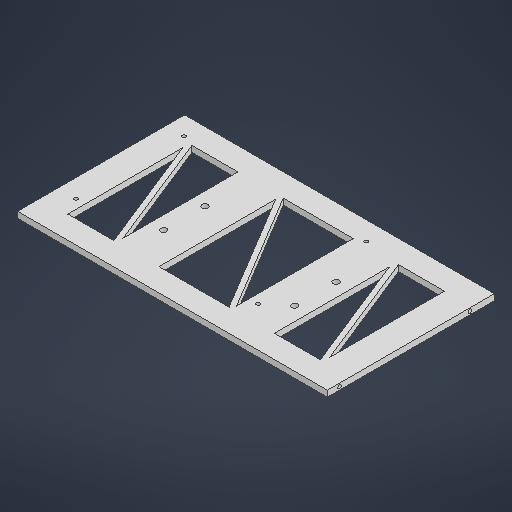
# Autodesk Inventor part: midplate
Saved by Autodesk Inventor 2025.1 (Build 291241000, 241)
## iProperties
Created: 2025-03-19
Part Number: midplate
Material: Generic
Document SubType Name: Modeling
Designer: m_kni
Density: 1 g/cm^3
Appearance: Default
Author: m_kni
## iProperties of the stored document midplate_3DPrint.ipt
Created: 2025-03-27
Part Number: midplate_3DPrint
Material: Generic
Document SubType Name: Modeling
Designer: jerem
Density: 1 g/cm^3
Appearance: Default
Author: jerem
Autodesk Inventor part; units mm, degrees
ref_plane "YZ Plane" through (0, 0, 0) normal (1, 0, 0) x (0, 1, 0)
ref_plane "XZ Plane" through (0, 0, 0) normal (0, 1, 0) x (-1, 0, 0)
ref_plane "XY Plane" through (0, 0, 0) normal (0, 0, 1) x (1, 0, 0)
sketch "Sketch1" plane through (0, 0, 0) normal (0, 1, 0) x (-1, 0, 0)
  circle A0 centre (-37.3734, -58.1709) radius 1.5
  circle A1 centre (112.6266, 30.8291) radius 1.5
  circle A2 centre (-37.3734, 30.8291) radius 1.5
  circle A3 centre (112.6266, -58.1709) radius 1.5
  circle A4 centre (54.1266, -16.9209) radius 2.5
  circle A5 centre (-53.8734, 17.0791) radius 2.5
  circle A6 centre (54.1266, 17.0791) radius 2.5
  circle A7 centre (-53.8734, -16.9209) radius 2.5
  line L0 (-127.3734, 73.8291) -> (127.6266, 73.8291)
  line L1 (-127.3734, -73.6709) -> (-127.3734, 73.8291)
  line L2 (127.6266, -73.6709) -> (-127.3734, -73.6709)
  line L3 (127.6266, 73.8291) -> (127.6266, -73.6709)
  point P0 (0, 0)
  point P1 (0.1266, 73.8291)
  constraints: 8 centre point, 8 end point
extrude "Extrusion1" add sketch "Sketch1" along normal blind 10
sketch "Sketch2" plane through (127.3734, 0, 73.8291) normal (1, 0, 0) x (0, 0, -1)
  line L0 (147.5, 0) -> (147.5, 10) projected
  line L1 (0, 0) -> (0, 10) projected
  circle A0 centre (127.5, 5) radius 1.5
  circle A1 centre (20, 5) radius 1.5
  point P0 (73.8291, 0)
  point P1 (0, 5)
  dimension "d2" = 20
  dimension "d3" = 20
  dimension "d4" = 3
  dimension "d5" = 3
  constraints: 2 centre point, 2 coincident, 1 midpoint
  measures "d2" distance from line of point (127.5, 5) L0
  measures "d3" distance of point (20, 5) point (0, 5)
  measures "d4" diameter of A0
  measures "d5" diameter of A1
extrude "Extrusion2" cut sketch "Sketch2" against normal blind 6
ref_plane "Work Plane1" through (-0.1266, 0, 73.8291) normal (1, 0, 0) x (0, 0, -1)
mirror "Mirror1" about plane through (-0.1266, 0, 73.8291) normal (1, 0, 0) of "Extrusion2"
sketch "Sketch3" plane through (-127.6266, 0, 73.8291) normal (0, 0, 1) x (1, 0, 0)
  line L0 (255, 10) -> (0, 10) projected
  line L1 (255, 0) -> (0, 0)
  line L2 (0, 0) -> (0, 10)
  line L3 (0, 10) -> (255, 10)
  line L4 (255, 10) -> (255, 0)
  point P0 (127.6266, 0)
  constraints: 8 end point, 2 parallel, 1 horizontal, 1 perpendicular
extrude "Extrusion3" cut sketch "Sketch3" against normal blind 10
sketch "Sketch4" plane through (0, 10, 0) normal (0, 1, 0) x (1, 0, 0)
  line L0 (127.3734, -63.8291) -> (127.3734, 73.6709) projected
  line L1 (-127.6266, -63.8291) -> (127.3734, -63.8291)
  line L2 (127.3734, -63.8291) -> (127.3734, 73.6709)
  line L3 (127.3734, 73.6709) -> (-127.6266, 73.6709)
  line L4 (-127.6266, 73.6709) -> (-127.6266, -63.8291)
  point P0 (0, 0)
  constraints: 8 end point, 2 parallel, 1 horizontal, 1 perpendicular
ref_plane "Work Plane2" through (0, 5, 0) normal (0, 1, 0) x (1, 0, 0)
extrude "Extrusion4" cut sketch "Sketch4" against normal blind 2.5
mirror "Mirror2" about plane through (0, 5, 0) normal (0, 1, 0) of "Extrusion4"
sketch "Sketch6" plane through (0, 7.5, 0) normal (0, 1, 0) x (1, 0, 0)
  circle A0 centre (37.3734, 58.1709) radius 1.5 projected
  circle A1 centre (-112.6266, -30.8291) radius 1.5 projected
  circle A2 centre (37.3734, -30.8291) radius 1.5 projected
  circle A3 centre (-112.6266, 58.1709) radius 1.5 projected
  circle A4 centre (-54.1266, 16.9209) radius 2.5 projected
  circle A5 centre (53.8734, -17.0791) radius 2.5 projected
  circle A6 centre (-54.1266, -17.0791) radius 2.5 projected
  circle A7 centre (53.8734, 16.9209) radius 2.5 projected
  line L0 (127.3734, 73.6709) -> (127.3734, -63.8291) projected
  line L1 (-127.6266, 73.6709) -> (127.3734, 73.6709) projected
  line L2 (-127.6266, -63.8291) -> (-127.6266, 73.6709) projected
  line L3 (127.3734, -63.8291) -> (-127.6266, -63.8291) projected
  line L4 (-30, 54.9209) -> (30, 54.9209)
  line L5 (30, 54.9209) -> (30, -45.0791)
  line L6 (30, -45.0791) -> (-30, -45.0791)
  line L7 (-30, -45.0791) -> (-30, 54.9209)
  line L8 (-105, 54.9209) -> (-65, 54.9209)
  line L9 (-65, 54.9209) -> (-65, -45.0791)
  line L10 (-65, -45.0791) -> (-105, -45.0791)
  line L11 (-105, -45.0791) -> (-105, 54.9209)
  line L12 (65, 54.9209) -> (105, 54.9209)
  line L13 (105, 54.9209) -> (105, -45.0791)
  line L14 (105, -45.0791) -> (65, -45.0791)
  line L15 (65, -45.0791) -> (65, 54.9209)
  line L16 (-65, 4.9209) -> (-30, 4.9209) construction
  line L17 (30, 4.9209) -> (65, 4.9209) construction
  line L18 (0, 0) -> (0, 54.9209) construction
  line L19 (0, 54.9209) -> (-0.1266, 73.6709) construction
  line L20 (0, -45.0791) -> (-0.1266, -63.8291) construction
  line L21 (-105, 54.9209) -> (-65, -45.0791) construction
  line L22 (-103.143, 55.6637) -> (-63.143, -44.3363)
  line L23 (-106.857, 54.1781) -> (-66.857, -45.8219)
  line L24 (-30, 54.9209) -> (30, -45.0791)
  line L25 (-31.715, 53.8919) -> (28.285, -46.1081)
  line L26 (-28.285, 55.9499) -> (31.715, -44.0501)
  line L27 (65, 54.9209) -> (105, -45.0791) construction
  line L28 (57.4212, 79.253) -> (105, -39.6939)
  line L29 (53.7073, 77.7675) -> (103.2874, -46.1827)
  point P0 (67.1541, 54.9209)
  point P1 (102.8459, -45.0791)
  point P2 (65, 49.5357)
  point P3 (-27.6676, 54.9209)
  point P4 (30, -41.1918)
  point P5 (27.6676, -45.0791)
  point P6 (-30, 51.0336)
  point P7 (-102.8459, 54.9209)
  point P8 (-65, -39.6939)
  point P9 (-67.1541, -45.0791)
  point P10 (-105, 49.5357)
  dimension "d12" = 60
  dimension "d13" = 100
  dimension "d14" = 40
  dimension "d15" = 35
  dimension "d16" = 2
  dimension "d17" = 2
  dimension "d18" = 2
  dimension "d19" = 2
  dimension "d20" = 2
  dimension "d21" = 2
  constraints: 52 end point, 12 parallel, 8 midpoint, 5 perpendicular, 4 equal length, 3 horizontal, 2 point on line, 1 collinear
  measures "d12" distance of L4.start L4.end
  measures "d13" distance of L6.end L4.start
  measures "d14" distance of L8.start L8.end
  measures "d15" distance of L16.start L16.end
  measures "d16" distance between parallel lines of L21 L23
  measures "d17" distance between parallel lines of L21 L22
  measures "d18" distance between parallel lines of L24 L25
  measures "d19" distance between parallel lines of L24 L26
  measures "d20" distance between parallel lines of L27 L29
  measures "d21" distance between parallel lines of L27 L28
extrude "Extrusion5" cut sketch "Sketch6" against normal through all contours L12 L13 L28 | L29 L14 L15 | L4 L5 L26 | L25 L6 L7 | L8 L9 L22 | L23 L10 L11
ref_plane "Work Plane3" through (0, 5, 0) normal (0, 1, 0) x (1, 0, 0)
equation "\"d17\" = d16"
equation "\"d18\" = d16"
equation "\"d19\" = d16"
equation "\"d20\" = d16"
equation "\"d21\" = d20"
body "Solid1"
